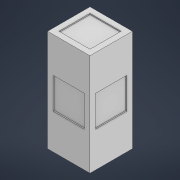
# Autodesk Inventor part: Shoulder_Cube_TestFit_V1
Saved by Autodesk Inventor 2022 (Build 260153000, 153)
## iProperties
Created: 2023-05-16
Part Number: Shoulder_Cube_TestFit_V1
Material: Generic
Document SubType Name: Modeling
Designer: Karl Spiteri
Density: 1 g/cm^3
Appearance: Default
Author: Karl Spiteri
Autodesk Inventor part; units mm, degrees
ref_plane "YZ Plane" through (0, 0, 0) normal (1, 0, 0) x (0, 1, 0)
ref_plane "XZ Plane" through (0, 0, 0) normal (0, 1, 0) x (-1, 0, 0)
ref_plane "XY Plane" through (0, 0, 0) normal (0, 0, 1) x (1, 0, 0)
sketch "Sketch1" plane through (0, 0, 0) normal (0, 0, 1) x (1, 0, 0)
  line L0 (0, 0) -> (-75, 0)
  line L1 (-75, 0) -> (-75, 180)
  line L2 (-75, 180) -> (0, 180)
  line L3 (0, 180) -> (0, 0)
  line L4 (-65, 170) -> (-10, 170)
  line L5 (-10, 10) -> (-65, 10)
  line L6 (-65, 10) -> (-65, 85)
  line L7 (-65, 95) -> (-65, 170)
  line L8 (-10, 170) -> (-10, 95)
  line L9 (-10, 85) -> (-10, 10)
  line L10 (-65, 85) -> (-65, 95)
  line L11 (-10, 95) -> (-10, 85)
  point P0 (-65, 90)
  point P1 (-10, 90)
  dimension "d35" = 75
  dimension "d36" = 180
  dimension "d37" = 55
  dimension "d38" = 160
  constraints: 24 end point, 3 parallel, 3 perpendicular, 2 horizontal, 2 midpoint, 1 collinear, 1 vertical
  measures "d35" distance of L1.end L2.end
  measures "d36" distance of L0.end L1.end
  measures "d37" distance of L5.start L5.end
  measures "d38" distance of L4.end L5.start
extrude "Extrusion7" add sketch "Sketch1" along normal blind 70
sketch "Sketch4" plane through (0, 0, 70) normal (0, 0, 1) x (1, 0, 0)
  line L0 (-75, 0) -> (0, 0) projected
  line L1 (0, 180) -> (-75, 180) projected
  line L2 (0, 0) -> (-75, 0)
  line L3 (-75, 0) -> (-75, 180)
  line L4 (-75, 180) -> (0, 180)
  line L5 (0, 180) -> (0, 0)
  constraints: 8 end point, 2 parallel, 1 horizontal, 1 perpendicular
extrude "Extrusion8" add sketch "Sketch4" along normal blind 5
sketch "Sketch5" plane through (0, 0, 75) normal (0, 0, 1) x (1, 0, 0)
  line L0 (-65, 85) -> (-65, 95)
  line L1 (-10, 95) -> (-10, 85)
  line L2 (-10, 62.5) -> (-10, 90)
  line L3 (-10, 62.5) -> (-65, 62.5)
  line L4 (-65, 62.5) -> (-65, 117.5)
  line L5 (-65, 117.5) -> (-10, 117.5)
  line L6 (-10, 117.5) -> (-10, 62.5)
  point P0 (-65, 90)
  dimension "d59" = 55
  dimension "d60" = 55
  constraints: 14 end point, 2 coincident, 2 midpoint, 2 parallel, 1 horizontal, 1 perpendicular, 1 vertical
  measures "d59" distance of L4.end L5.end
  measures "d60" distance of L3.end L4.end
extrude "Extrusion9" cut sketch "Sketch5" against normal blind 2
sketch "Sketch6" plane through (0, 0, 0) normal (1, 0, 0) x (0, 0, -1)
  line L0 (-10, 62.5) -> (-65, 62.5)
  line L1 (-65, 62.5) -> (-65, 117.5)
  line L2 (-65, 117.5) -> (-10, 117.5)
  line L3 (-10, 117.5) -> (-10, 62.5)
  dimension "d67" = 55
  dimension "d68" = 55
  constraints: 8 end point, 2 parallel, 1 horizontal, 1 perpendicular
  measures "d67" distance of L1.end L2.end
  measures "d68" distance of L0.end L1.end
extrude "Extrusion10" cut sketch "Sketch6" against normal blind 2
sketch "Sketch7" plane through (-75, 0, 0) normal (-1, 0, 0) x (0, 0, 1)
  line L0 (10, 62.5) -> (65, 62.5) projected
  line L1 (10, 62.5) -> (65, 62.5)
  line L2 (65, 62.5) -> (65, 117.5)
  line L3 (65, 117.5) -> (10, 117.5)
  line L4 (10, 117.5) -> (10, 62.5)
  point P0 (0, 0)
  dimension "d71" = 55
  dimension "d72" = 55
  constraints: 8 end point, 2 parallel, 1 horizontal, 1 perpendicular
  measures "d71" distance of L3.end L2.end
  measures "d72" distance of L2.end L1.end
extrude "Extrusion11" cut sketch "Sketch7" against normal blind 2
sketch "Sketch8" plane through (-75, 0, 0) normal (0, -1, 0) x (1, 0, 0)
  line L0 (10, 10) -> (65, 10)
  line L1 (65, 10) -> (65, 65)
  line L2 (65, 65) -> (10, 65)
  line L3 (10, 65) -> (10, 10)
  point P0 (75, 0)
  dimension "d75" = 55
  dimension "d76" = 55
  constraints: 8 end point, 2 parallel, 1 horizontal, 1 perpendicular
  measures "d75" distance of L2.end L1.end
  measures "d76" distance of L1.end L0.end
extrude "Extrusion12" cut sketch "Sketch8" against normal blind 2
sketch "Sketch9" plane through (-75, 180, 0) normal (0, 1, 0) x (1, 0, 0)
  line L0 (10, -10) -> (65, -10)
  line L1 (65, -10) -> (65, -65)
  line L2 (65, -65) -> (10, -65)
  line L3 (10, -65) -> (10, -10)
  point P0 (75, 0)
  dimension "d79" = 55
  dimension "d80" = 55
  constraints: 8 end point, 2 parallel, 1 horizontal, 1 perpendicular
  measures "d79" distance of L1.end L2.end
  measures "d80" distance of L0.end L1.end
extrude "Extrusion13" cut sketch "Sketch9" against normal blind 2
body "Solid5"
